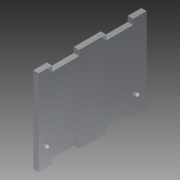
# Autodesk Inventor part: Side
Saved by Autodesk Inventor 2015 (Build 190159000, 159)
## iProperties
Created: 2017-03-04
Part Number: Side
Material: Generic
Document SubType Name: Modeling
Designer: Guy
Density: 1 g/cm^3
Appearance: Default
Author: Guy
Autodesk Inventor part; units mm, degrees
ref_plane "YZ Plane" through (0, 0, 0) normal (1, 0, 0) x (0, 1, 0)
ref_plane "XZ Plane" through (0, 0, 0) normal (0, 1, 0) x (-1, 0, 0)
ref_plane "XY Plane" through (0, 0, 0) normal (0, 0, 1) x (1, 0, 0)
sketch "Sketch1" plane through (0, 0, 0) normal (1, 0, 0) x (0, 1, 0)
  line L0 (0, 0) -> (120, 0)
  line L1 (120, 0) -> (120, -95)
  line L2 (120, -95) -> (0, -95)
  line L3 (0, -95) -> (0, 0)
  dimension "d0" = 120
  dimension "d1" = 95
  constraints: 8 end point, 2 parallel, 1 horizontal, 1 perpendicular
  measures "d0" distance of L1.end L2.end
  measures "d1" distance of L0.end L1.end
extrude "Extrusion1" add sketch "Sketch1" along normal blind 6
sketch "Sketch2" plane through (6, 0, 0) normal (1, 0, 0) x (0, 0, -1)
  line L0 (0, 120) -> (0, 0) projected
  line L1 (0, 0) -> (95, 0) projected
  line L2 (95, 0) -> (95, 120) projected
  line L3 (95, 120) -> (0, 120) projected
  line L4 (0, 120) -> (0, 0) projected
  line L5 (0, 15) -> (5.875, 15)
  line L6 (5.875, 15) -> (5.875, 45)
  line L7 (5.875, 45) -> (0, 45)
  line L8 (0, 45) -> (0, 15)
  line L9 (0, 75) -> (5.875, 75)
  line L10 (5.875, 75) -> (5.875, 105)
  line L11 (5.875, 105) -> (0, 105)
  line L12 (0, 105) -> (0, 75)
  line L13 (95, 15) -> (89.125, 15)
  line L14 (89.125, 15) -> (89.125, 45)
  line L15 (89.125, 45) -> (95, 45)
  line L16 (95, 45) -> (95, 15)
  line L17 (95, 75) -> (89.125, 75)
  line L18 (89.125, 75) -> (89.125, 105)
  line L19 (89.125, 105) -> (95, 105)
  line L20 (95, 105) -> (95, 75)
  line L21 (-12.0657, 60) -> (104.2665, 60)
  line L22 (95, 120) -> (0, 120) projected
  dimension "d5" = 5.875
  dimension "d6" = 5.875
  dimension "d8" = 30
  dimension "d9" = 30
  dimension "d22" = 60
  dimension "d23" = 15
  dimension "d24" = 15
  constraints: 34 end point, 9 parallel, 5 collinear, 5 horizontal, 5 point on line, 4 perpendicular
  measures "d5" distance between parallel lines of L10 L0
  measures "d6" distance between parallel lines of L20 L18
  measures "d8" distance between parallel lines of L19 L17
  measures "d9" distance between parallel lines of L13 L15
  measures "d22" distance between parallel lines of L21 L3
  measures "d23" distance between parallel lines of L17 L21
  measures "d24" distance between parallel lines of L15 L21
extrude "Extrusion2" cut sketch "Sketch2" against normal up to next contours L11 L10 L9 L0 | L2 L17 L18 L19 | L7 L6 L5 L0 | L2 L13 L14 L15
sketch "Sketch3" plane through (6, 0, 0) normal (1, 0, 0) x (0, 0, -1)
  circle A0 centre (75, 10) radius 2.5
  circle A1 centre (75, 110) radius 2.5
  line L0 (95, 105) -> (95, 120) projected
  line L1 (95, 120) -> (0, 120) projected
  line L2 (95, 0) -> (95, 15) projected
  line L3 (0, 0) -> (95, 0) projected
  dimension "d13" = 20
  dimension "d14" = 10
  dimension "d15" = 5
  dimension "d17" = 10
  dimension "d18" = 20
  dimension "d19" = 5
  constraints: 2 centre point
  measures "d13" distance from line of L0 A1.centre
  measures "d14" distance from line of A1.centre L1
  measures "d15" diameter of A1
  measures "d17" distance from line of A0.centre L3
  measures "d18" distance from line of A0.centre L2
  measures "d19" diameter of A0
extrude "Extrusion3" cut sketch "Sketch3" against normal up to next
body "Solid1"
